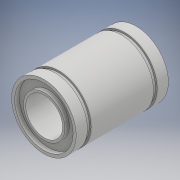
# Autodesk Inventor part: rolamento_linear_lm16uu.iam
Saved by Autodesk Inventor 2018 (Build 220112000, 112)
## iProperties
Created: 2018-05-16
Part Number: rolamento_linear_lm16uu.iam
Material: Genérico
Document SubType Name: Modeling
Designer: Usuario
Density: 1 g/cm^3
Appearance: Padrão
Mass: 6.471 g
Surface Area: 72.2059 cm^2
Volume: 6.471 cm^3
Author: Usuario
Autodesk Inventor part; units mm, degrees
ref_plane "YZ Plane" through (0, 0, 0) normal (1, 0, 0) x (0, 1, 0)
ref_plane "XZ Plane" through (0, 0, 0) normal (0, 1, 0) x (-1, 0, 0)
ref_plane "XY Plane" through (0, 0, 0) normal (0, 0, 1) x (1, 0, 0)
sketch "Esboço1" plane through (0, 0, 0) normal (0, 0, 1) x (1, 0, 0)
  line L0 (-10.5, 0) -> (-10.5, 3.65)
  line L1 (-10.5, 3.65) -> (-9.95, 3.65)
  line L2 (-9.95, 3.65) -> (-9.95, 4.85)
  line L3 (-9.95, 4.85) -> (-10.5, 4.85)
  line L4 (-10.5, 4.85) -> (-10.5, 25.15)
  line L5 (-10.5, 25.15) -> (-9.95, 25.15)
  line L6 (-9.95, 25.15) -> (-9.95, 26.35)
  line L7 (-9.95, 26.35) -> (-10.5, 26.35)
  line L8 (-10.5, 26.35) -> (-10.5, 30)
  line L9 (-10.5, 30) -> (-9.5, 30)
  line L10 (-10.5, 0) -> (-9.5, 0)
  line L11 (-9.5, 0) -> (0, 0) construction
  line L12 (0, 0) -> (0, 30) construction
  line L13 (0, 30) -> (-9.5, 30) construction
  line L14 (-9.5, 30) -> (-9.5, 0)
  dimension "d0" = 9.5
  dimension "d1" = 30
  dimension "d2" = 3.65
  dimension "d3" = 3.65
  dimension "d4" = 0.55
  dimension "d5" = 1.2
  dimension "d6" = 1.2
  dimension "d8" = 1
  constraints: 30 end point, 9 perpendicular, 6 point on line, 2 horizontal
  measures "d0" distance of L12.end L9.end
  measures "d1" distance of L0.start L8.end
  measures "d2" distance from line of L7 L8.end
  measures "d3" distance between parallel lines of L10 L1
  measures "d4" distance between parallel lines of L6 L4
  measures "d5" distance of L5.end L6.end
  measures "d6" distance of L1.end L2.end
  measures "d8" distance of L8.end L9.end
sketch "Esboço3" plane through (0, 0, 0) normal (0, 0, 1) x (1, 0, 0)
  line L0 (0, 0) -> (-6, 0) construction
  line L1 (-6, 0) -> (-6, 30) construction
  line L2 (-6, 30) -> (0, 30) construction
  line L3 (0, 30) -> (0, 0) construction
  line L4 (0, 30) -> (0, 28.5) construction
  line L5 (0, 0) -> (0, 1.5) construction
  line L6 (0, 1.5) -> (-9.49, 1.5) construction
  line L7 (-9.49, 28.5) -> (-6.76, 28.5)
  line L8 (-6, 28.5) -> (-6, 29.9)
  line L9 (-6, 29.9) -> (-6.76, 29.9)
  line L10 (-6.76, 29.9) -> (-6.76, 28.5)
  line L11 (-9.49, 1.5) -> (-6.76, 1.5)
  line L12 (-6, 1.5) -> (-6, 0.1)
  line L13 (-6, 0.1) -> (-6.76, 0.1)
  line L14 (-6.76, 0.1) -> (-6.76, 1.5)
  line L15 (0, 28.5) -> (-6, 28.5) construction
  line L16 (-6.76, 28.5) -> (-9.49, 28.5) construction
  line L17 (-6, 28.5) -> (-6, 1.5)
  line L18 (-9.49, 1.5) -> (-9.49, 28.5)
  dimension "d11" = 6
  dimension "d14" = 1.5
  dimension "d16" = 1.5
  dimension "d18" = 1.4
  dimension "d19" = 0.76
  dimension "d20" = 1.4
  dimension "d21" = 0.76
  dimension "d22" = 3.49
  constraints: 38 end point, 10 perpendicular, 9 point on line, 1 horizontal
  measures "d11" distance of L0.start L0.end
  measures "d14" distance of L2.end L4.end
  measures "d16" distance of L0.start L5.end
  measures "d18" distance of L8.start L8.end
  measures "d19" distance of L8.end L9.end
  measures "d20" distance of L12.start L12.end
  measures "d21" distance of L12.end L13.end
  measures "d22" distance between parallel lines of L18 L17
revolve "Revolução1" add sketch "Esboço3" angle 360 about axis through (0, 30, 0) along (0, -1, 0)
revolve "Revolução2" add sketch "Esboço1" angle 360 about axis through (0, 0, 0) along (0, 1, 0)
